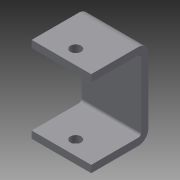
# Autodesk Inventor part: pulley mount. actual ipt
Saved by Autodesk Inventor 2013 (Build 170138000, 138)
## iProperties
Created: 2013-01-31
Part Number: pulley mount. actual ipt
Material: Generic
Document SubType Name: Sheet Metal
Designer: Arpan
Density: 1 g/cm^3
Sheet Metal Rule: Default
Author: Arpan
Autodesk Inventor part; units mm, degrees
ref_plane "YZ Plane" through (0, 0, 0) normal (1, 0, 0) x (0, 1, 0)
ref_plane "XZ Plane" through (0, 0, 0) normal (0, 1, 0) x (-1, 0, 0)
ref_plane "XY Plane" through (0, 0, 0) normal (0, 0, 1) x (1, 0, 0)
sketch "Sketch1" plane through (0, 0, 0) normal (0, 0, 1) x (1, 0, 0)
  circle A0 centre (5.881, 13.6671) radius 3.1287
  circle A1 centre (20.5836, 13.6671) radius 3.1287
  line L0 (0, -0.9379) -> (26.4647, -0.9379)
  line L1 (26.4647, 28.2721) -> (26.4647, -0.9379)
  line L2 (0, 28.2721) -> (26.4647, 28.2721)
  line L3 (0, -0.9379) -> (0, 28.2721)
  point P0 (0, 0)
  dimension "d4" = 14.7026
  dimension "d5" = 29.21
  dimension "d21" = 14.605
  measures "d4" distance of A0.centre A1.centre
  measures "d5" distance of L1.start L0.end
  measures "d21" distance from line of L2 A0.centre
extrude "Plate1" add sketch "Sketch1" along normal blind 3.175 contours A0 | A1 | L3 L2 L1 L0
sketch "Sketch2" plane through (0, 29.5421, 4.445) normal (0, 1, 0) x (-1, 0, 0)
  line L0 (-26.4647, 0) -> (0, 0)
  line L1 (0, 0) -> (0, 20.955)
  line L2 (0, 20.955) -> (-26.4647, 20.955)
  line L3 (-26.4647, 20.955) -> (-26.4647, 0)
  constraints: 6 end point, 1 horizontal, 1 perpendicular, 1 vertical
edge flange "Flange1" height 25.4 angle 90 thickness 3.175 bend radius 1.27 thickness toward (0, 1, 0) relief tear relief width 3.175 relief depth 1.5875 corner gap 3.175 corner form 0 edges at (13.2323, 28.2721, 3.175) (13.2323, -0.9379, 3.175) wall of the first edge with corners at (26.4647, 29.5421, 4.445) (0, 29.5421, 4.445) (0, 29.5421, 25.4) (26.4647, 29.5421, 25.4)
bend "Bend1"
corner "Corner1"
sketch "Sketch3" plane through (0, 32.7171, 25.4) normal (0, 1, 0) x (1, 0, 0)
  line L0 (26.4647, 0) -> (0, 0) projected
  line L1 (26.4647, 20.955) -> (26.4647, 0) projected
  line L2 (13.2323, 0) -> (13.2323, 6.35)
  circle A0 centre (13.2323, 6.35) radius 2.3813
  point P0 (0, 25.4)
  dimension "d17" = 6.35
  dimension "d18" = 4.7625
  constraints: 2 end point, 1 centre point, 1 coincident, 1 midpoint, 1 parallel
  measures "d17" distance of L2.start L2.end
  measures "d18" diameter of A0
extrude "Extrusion1" cut sketch "Sketch3" against normal blind 76174.6
equation "\"d7\" = BendReliefWidth"
equation "\"d8\" = BendReliefDepth"
equation "\"d9\" = MinimumRemnant"
equation "\"d10\" = BendRadius"
equation "\"d14\" = CornerReliefSize"
equation "\"d15\" = GapSize"
equation "\"d16\" = JacobiRadiusSize"
equation "\"BendRadius\" = Thickness"
equation "\"BendReliefWidth\" = Thickness"
equation "\"BendReliefDepth\" = 0.5 * Thickness"
equation "\"CornerReliefSize\" = 4 * Thickness"
equation "\"MinimumRemnant\" = 2 * Thickness"
equation "\"TransitionRadius\" = BendRadius"
equation "\"JacobiRadiusSize\" = Thickness"
equation "\"GapSize\" = Thickness"
equation "\"d6\" = BendRadius"
equation "\"Thickness\" = 3.175"
body "Solid1"
